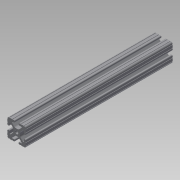
# Autodesk Inventor part: 1515
Saved by Autodesk Inventor 2013 (Build 170138000, 138)
## iProperties
Created: 2014-04-23
Part Number: 1515
Material: Generic
Document SubType Name: Modeling
Density: 1 g/cm^3
Vendor: 80/20 Inc.
Engineer: Ross Bowman
Designer: Ross Bowman
Catalog Web Link: 8020.net
Company: 80/20 Inc.
Author: Ross Bowman
Keywords: 80/20 , 8020 , T-Slot , Extrusion
Material: 6105-T5 Aluminum
Autodesk Inventor part; units mm, degrees
ref_plane "YZ Plane" through (0, 0, 0) normal (1, 0, 0) x (0, 1, 0)
ref_plane "XZ Plane" through (0, 0, 0) normal (0, 1, 0) x (-1, 0, 0)
ref_plane "XY Plane" through (0, 0, 0) normal (0, 0, 1) x (1, 0, 0)
sketch "Sketch1" plane through (0, 0, 0) normal (0, 0, 1) x (1, 0, 0)
  circle A0 centre (0, 0) radius 3.3274
  arc A1 (-10.287, 13.5524) -> (-10.0229, 12.9148) centre (-9.3853, 13.5524) ccw
  line L0 (-10.287, 13.5524) -> (-10.287, 14.0843)
  arc A2 (-9.3853, 14.986) -> (-10.287, 14.0843) centre (-9.3853, 14.0843) ccw
  line L1 (-9.3853, 14.986) -> (-5.6176, 14.986)
  arc A3 (-5.6176, 14.986) -> (-4.064, 16.5396) centre (-5.6176, 16.5396) ccw
  line L2 (-4.064, 16.5396) -> (-4.064, 17.4964)
  arc A4 (-4.064, 17.4964) -> (-5.6176, 19.05) centre (-5.6176, 17.4964) ccw
  line L3 (-5.6176, 19.05) -> (-7.9742, 19.05)
  arc A5 (-9.4982, 19.05) -> (-7.9742, 19.05) centre (-8.7362, 19.05) ccw
  line L4 (-9.4982, 19.05) -> (-14.3277, 19.05)
  arc A6 (-15.8475, 19.05) -> (-14.3277, 19.05) centre (-15.0876, 18.9933) ccw
  arc A7 (-15.8475, 19.05) -> (-19.05, 15.8475) centre (-15.8751, 15.8751) ccw
  arc A8 (-19.05, 14.3277) -> (-19.05, 15.8475) centre (-18.9933, 15.0876) ccw
  line L5 (-19.05, 14.3277) -> (-19.05, 9.4961)
  arc A9 (-19.05, 7.9763) -> (-19.05, 9.4961) centre (-18.9933, 8.7362) ccw
  line L6 (-19.05, 7.9763) -> (-19.05, 5.6176)
  arc A10 (-19.05, 5.6176) -> (-17.4964, 4.064) centre (-17.4964, 5.6176) ccw
  line L7 (-17.4964, 4.064) -> (-16.5396, 4.064)
  arc A11 (-16.5396, 4.064) -> (-14.986, 5.6176) centre (-16.5396, 5.6176) ccw
  line L8 (-14.986, 5.6176) -> (-14.986, 9.3853)
  arc A12 (-14.0843, 10.287) -> (-14.986, 9.3853) centre (-14.0843, 9.3853) ccw
  line L9 (-14.0843, 10.287) -> (-13.516, 10.287)
  arc A13 (-12.8784, 10.0229) -> (-13.516, 10.287) centre (-13.516, 9.3853) ccw
  line L10 (-12.8784, 10.0229) -> (-8.1476, 5.2921)
  arc A14 (-6.7564, 1.9335) -> (-8.1476, 5.2921) centre (-11.5062, 1.9335) ccw
  line L11 (-6.7564, 1.9335) -> (-6.7564, -1.9335)
  arc A15 (-8.1476, -5.2921) -> (-6.7564, -1.9335) centre (-11.5062, -1.9335) ccw
  line L12 (-8.1476, -5.2921) -> (-12.8784, -10.0229)
  arc A16 (-13.516, -10.287) -> (-12.8784, -10.0229) centre (-13.516, -9.3853) ccw
  line L13 (-13.516, -10.287) -> (-14.0843, -10.287)
  arc A17 (-14.986, -9.3853) -> (-14.0843, -10.287) centre (-14.0843, -9.3853) ccw
  line L14 (-14.986, -9.3853) -> (-14.986, -5.6176)
  arc A18 (-14.986, -5.6176) -> (-16.5396, -4.064) centre (-16.5396, -5.6176) ccw
  line L15 (-16.5396, -4.064) -> (-17.4964, -4.064)
  arc A19 (-17.4964, -4.064) -> (-19.05, -5.6176) centre (-17.4964, -5.6176) ccw
  line L16 (-19.05, -5.6176) -> (-19.05, -7.9763)
  arc A20 (-19.05, -9.4961) -> (-19.05, -7.9763) centre (-18.9933, -8.7362) ccw
  line L17 (-19.05, -9.4961) -> (-19.05, -14.3277)
  arc A21 (-19.05, -15.8475) -> (-19.05, -14.3277) centre (-18.9933, -15.0876) ccw
  arc A22 (-19.05, -15.8475) -> (-15.8475, -19.05) centre (-15.8751, -15.8751) ccw
  arc A23 (-14.3277, -19.05) -> (-15.8475, -19.05) centre (-15.0876, -18.9933) ccw
  line L18 (-14.3277, -19.05) -> (-9.4961, -19.05)
  arc A24 (-7.9763, -19.05) -> (-9.4961, -19.05) centre (-8.7362, -18.9933) ccw
  line L19 (-7.9763, -19.05) -> (-5.6176, -19.05)
  arc A25 (-5.6176, -19.05) -> (-4.064, -17.4964) centre (-5.6176, -17.4964) ccw
  line L20 (-4.064, -17.4964) -> (-4.064, -16.5396)
  arc A26 (-4.064, -16.5396) -> (-5.6176, -14.986) centre (-5.6176, -16.5396) ccw
  line L21 (-5.6176, -14.986) -> (-9.3853, -14.986)
  arc A27 (-10.287, -14.0843) -> (-9.3853, -14.986) centre (-9.3853, -14.0843) ccw
  line L22 (-10.287, -14.0843) -> (-10.287, -13.5524)
  arc A28 (-10.0229, -12.9148) -> (-10.287, -13.5524) centre (-9.3853, -13.5524) ccw
  line L23 (-10.0229, -12.9148) -> (-5.2522, -8.144)
  arc A29 (-1.9022, -6.7564) -> (-5.2522, -8.144) centre (-1.9022, -11.494) ccw
  line L24 (-1.9022, -6.7564) -> (1.9022, -6.7564)
  arc A30 (5.2522, -8.144) -> (1.9022, -6.7564) centre (1.9022, -11.494) ccw
  line L25 (5.2522, -8.144) -> (10.0229, -12.9148)
  arc A31 (10.287, -13.5524) -> (10.0229, -12.9148) centre (9.3853, -13.5524) ccw
  line L26 (10.287, -13.5524) -> (10.287, -14.0843)
  arc A32 (9.3853, -14.986) -> (10.287, -14.0843) centre (9.3853, -14.0843) ccw
  line L27 (9.3853, -14.986) -> (5.6176, -14.986)
  arc A33 (5.6176, -14.986) -> (4.064, -16.5396) centre (5.6176, -16.5396) ccw
  line L28 (4.064, -16.5396) -> (4.064, -17.4964)
  arc A34 (4.064, -17.4964) -> (5.6176, -19.05) centre (5.6176, -17.4964) ccw
  line L29 (5.6176, -19.05) -> (7.9763, -19.05)
  arc A35 (9.4961, -19.05) -> (7.9763, -19.05) centre (8.7362, -18.9933) ccw
  line L30 (9.4961, -19.05) -> (14.3277, -19.05)
  arc A36 (15.8475, -19.05) -> (14.3277, -19.05) centre (15.0876, -18.9933) ccw
  arc A37 (15.8475, -19.05) -> (19.05, -15.8475) centre (15.8751, -15.8751) ccw
  arc A38 (19.05, -14.3277) -> (19.05, -15.8475) centre (18.9933, -15.0876) ccw
  line L31 (19.05, -14.3277) -> (19.05, -9.4961)
  arc A39 (19.05, -7.9763) -> (19.05, -9.4961) centre (18.9933, -8.7362) ccw
  line L32 (19.05, -7.9763) -> (19.05, -5.6176)
  arc A40 (19.05, -5.6176) -> (17.4964, -4.064) centre (17.4964, -5.6176) ccw
  line L33 (17.4964, -4.064) -> (16.5396, -4.064)
  arc A41 (16.5396, -4.064) -> (14.986, -5.6176) centre (16.5396, -5.6176) ccw
  line L34 (14.986, -5.6176) -> (14.986, -9.3853)
  arc A42 (14.0843, -10.287) -> (14.986, -9.3853) centre (14.0843, -9.3853) ccw
  line L35 (14.0843, -10.287) -> (13.516, -10.287)
  arc A43 (12.8784, -10.0229) -> (13.516, -10.287) centre (13.516, -9.3853) ccw
  line L36 (12.8784, -10.0229) -> (8.1476, -5.2921)
  arc A44 (6.7564, -1.9335) -> (8.1476, -5.2921) centre (11.5062, -1.9335) ccw
  line L37 (6.7564, -1.9335) -> (6.7564, 1.9335)
  arc A45 (8.1476, 5.2921) -> (6.7564, 1.9335) centre (11.5062, 1.9335) ccw
  line L38 (8.1476, 5.2921) -> (12.8784, 10.0229)
  arc A46 (13.516, 10.287) -> (12.8784, 10.0229) centre (13.516, 9.3853) ccw
  line L39 (13.516, 10.287) -> (14.0843, 10.287)
  arc A47 (14.986, 9.3853) -> (14.0843, 10.287) centre (14.0843, 9.3853) ccw
  line L40 (14.986, 9.3853) -> (14.986, 5.6176)
  arc A48 (14.986, 5.6176) -> (16.5396, 4.064) centre (16.5396, 5.6176) ccw
  line L41 (16.5396, 4.064) -> (17.4964, 4.064)
  arc A49 (17.4964, 4.064) -> (19.05, 5.6176) centre (17.4964, 5.6176) ccw
  line L42 (19.05, 5.6176) -> (19.05, 7.9763)
  arc A50 (19.05, 9.4961) -> (19.05, 7.9763) centre (18.9933, 8.7362) ccw
  line L43 (19.05, 9.4961) -> (19.05, 14.3277)
  arc A51 (19.05, 15.8475) -> (19.05, 14.3277) centre (18.9933, 15.0876) ccw
  arc A52 (19.05, 15.8475) -> (15.8475, 19.05) centre (15.8751, 15.8751) ccw
  arc A53 (14.3277, 19.05) -> (15.8475, 19.05) centre (15.0876, 18.9933) ccw
  line L44 (14.3277, 19.05) -> (9.4982, 19.05)
  arc A54 (7.9742, 19.05) -> (9.4982, 19.05) centre (8.7362, 19.05) ccw
  line L45 (7.9742, 19.05) -> (5.6176, 19.05)
  arc A55 (5.6176, 19.05) -> (4.064, 17.4964) centre (5.6176, 17.4964) ccw
  line L46 (4.064, 17.4964) -> (4.064, 16.5396)
  arc A56 (4.064, 16.5396) -> (5.6176, 14.986) centre (5.6176, 16.5396) ccw
  line L47 (5.6176, 14.986) -> (9.3853, 14.986)
  arc A57 (10.287, 14.0843) -> (9.3853, 14.986) centre (9.3853, 14.0843) ccw
  line L48 (10.287, 14.0843) -> (10.287, 13.5524)
  arc A58 (10.0229, 12.9148) -> (10.287, 13.5524) centre (9.3853, 13.5524) ccw
  line L49 (10.0229, 12.9148) -> (5.2522, 8.144)
  arc A59 (1.9022, 6.7564) -> (5.2522, 8.144) centre (1.9022, 11.494) ccw
  line L50 (1.9022, 6.7564) -> (-1.9022, 6.7564)
  arc A60 (-5.2522, 8.144) -> (-1.9022, 6.7564) centre (-1.9022, 11.494) ccw
  line L51 (-5.2522, 8.144) -> (-10.0229, 12.9148)
  constraints: 120 point on circle, 104 end point, 61 centre point
extrude "Extrusion1" add sketch "Sketch1" against normal blind 304.8
body "Solid1"
